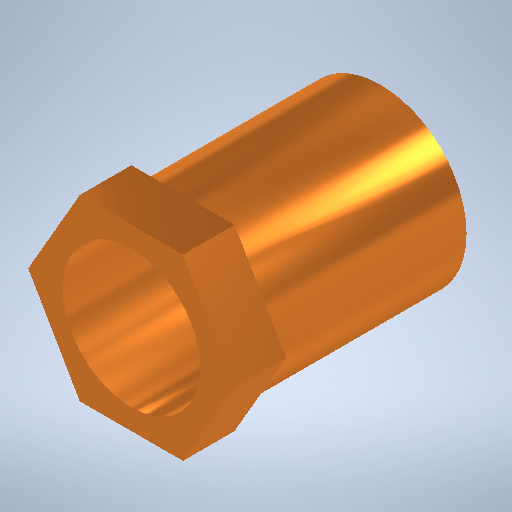
# Autodesk Inventor part: überwurfmutter
Saved by Autodesk Inventor 2025 (Build 290162010, 162A)
## iProperties
Created: 2024-04-30
Part Number: überwurfmutter
Material: Gold
Document SubType Name: Modeling
Designer: ffogue
Density: 19.3 g/cm^3
Appearance: Metal 1600F Hot
Author: ffogue
Autodesk Inventor part; units mm, degrees
ref_plane "YZ Plane" through (0, 0, 0) normal (1, 0, 0) x (0, 1, 0)
ref_plane "XZ Plane" through (0, 0, 0) normal (0, 1, 0) x (-1, 0, 0)
ref_plane "XY Plane" through (0, 0, 0) normal (0, 0, 1) x (1, 0, 0)
sketch "Skizze1" plane through (0, 0, 0) normal (0, 1, 0) x (-1, 0, 0)
  line L0 (6, 0) -> (3, -5.1962)
  line L1 (3, -5.1962) -> (-3, -5.1962)
  line L2 (-3, -5.1962) -> (-6, 0)
  line L3 (-6, 0) -> (-3, 5.1962)
  line L4 (-3, 5.1962) -> (3, 5.1962)
  line L5 (3, 5.1962) -> (6, 0)
  point P0 (0, 0)
  point P1 (0, 0)
  dimension "d5" = 12
  constraints: 12 end point, 1 coincident, 1 horizontal alignment, 13 other
  measures "d5" distance of L2.end L0.start
extrude "Extrusion3" add sketch "Skizze1" along normal blind 3
sketch "Sketch4" plane through (0, 3, 0) normal (0, 1, 0) x (1, 0, 0)
  circle A0 centre (0, 0) radius 5
  dimension "d12" = 10
  constraints: 1 centre point, 1 coincident
  measures "d12" diameter of A0
extrude "Extrusion4" add sketch "Sketch4" along normal blind 11.5
sketch "Sketch5" plane through (0, 14.5, 0) normal (0, 1, 0) x (1, 0, 0)
  circle A0 centre (0, 0) radius 5 construction
  constraints: 1 coincident
hole "Hole1" at (0, 14.5, 0) direction (0, -1, 0) diameter 8 depth 14.5
body "Solid2"
